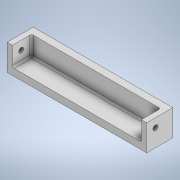
# Autodesk Inventor part: leg_8
Saved by Autodesk Inventor 2021.3 (Build 253353010, 353A)
## iProperties
Created: 2021-10-20
Part Number: leg_8
Material: Generic
Document SubType Name: Modeling
Designer: jesse
Density: 1 g/cm^3
Appearance: Default
Author: jesse
Autodesk Inventor part; units mm, degrees
ref_plane "YZ Plane" through (0, 0, 0) normal (1, 0, 0) x (0, 1, 0)
ref_plane "XZ Plane" through (0, 0, 0) normal (0, 1, 0) x (-1, 0, 0)
ref_plane "XY Plane" through (0, 0, 0) normal (0, 0, 1) x (1, 0, 0)
sketch "Sketch1" plane through (0, 0, 0) normal (0, 1, 0) x (-1, 0, 0)
  line L0 (39.5855, 7.487) -> (-40.4145, 7.487)
  line L1 (-40.4145, 7.487) -> (-40.4145, -7.513)
  line L2 (-40.4145, -7.513) -> (39.5855, -7.513)
  line L3 (39.5855, -7.513) -> (39.5855, 7.487)
  point P0 (0, 0)
  dimension "d0" = 80
  dimension "d1" = 15
  constraints: 8 end point, 2 parallel, 1 horizontal, 1 perpendicular
  measures "d0" distance of L1.end L2.end
  measures "d1" distance of L2.end L0.start
extrude "Extrusion1" add sketch "Sketch1" along normal blind 15
sketch "Sketch2" plane through (0, 15, 0) normal (0, 1, 0) x (1, 0, 0)
  line L0 (-39.5855, -7.487) -> (40.4145, -7.487) projected
  line L1 (-36.5855, -7.487) -> (37.4145, -7.487)
  line L2 (37.4145, -7.487) -> (37.4145, 3.513)
  line L3 (37.4145, 3.513) -> (-36.5855, 3.513)
  line L4 (-36.5855, 3.513) -> (-36.5855, -7.487)
  line L5 (40.4145, 7.513) -> (-39.5855, 7.513) projected
  line L6 (-39.5855, 7.513) -> (-39.5855, -7.487) projected
  line L7 (40.4145, -7.487) -> (40.4145, 7.513) projected
  point P0 (0, 0)
  point P1 (37.4145, -7.487)
  dimension "d4" = 4
  dimension "d5" = 3
  dimension "d6" = 3
  constraints: 8 end point, 2 parallel, 1 horizontal, 1 perpendicular, 1 point on line
  measures "d4" distance between parallel lines of L3 L5
  measures "d5" distance between parallel lines of L4 L6
  measures "d6" distance between parallel lines of L7 L2
extrude "Extrusion2" cut sketch "Sketch2" against normal blind 11 contours L4 L3 L2 L0
sketch "Sketch3" plane through (-39.5855, 0, -7.513) normal (-1, 0, 0) x (0, 0, 1)
  circle A0 centre (10, 10) radius 1.4
  line L0 (15, 4) -> (4, 4) projected
  line L1 (4, 15) -> (4, 4) projected
  point P0 (7.513, 0)
  dimension "d9" = 2.8
  dimension "d10" = 6
  dimension "d11" = 6
  constraints: 1 centre point
  measures "d9" diameter of A0
  measures "d10" distance from line of L0 A0.centre
  measures "d11" distance from line of L1 A0.centre
extrude "Extrusion3" cut sketch "Sketch3" against normal through all
fillet "Fillet1" radius 1 1 edges at (0.4145, 4, -3.513)
fillet "Fillet2" radius 1 3 edges at (-36.5855, 10, -3.513) (-36.5855, 4.2929, -3.2201) (-36.5855, 4, 2.487)
fillet "Fillet3" radius 1 3 edges at (37.4145, 4, 2.487) (37.4145, 4.2929, -3.2201) (37.4145, 10, -3.513)
body "Solid1"
